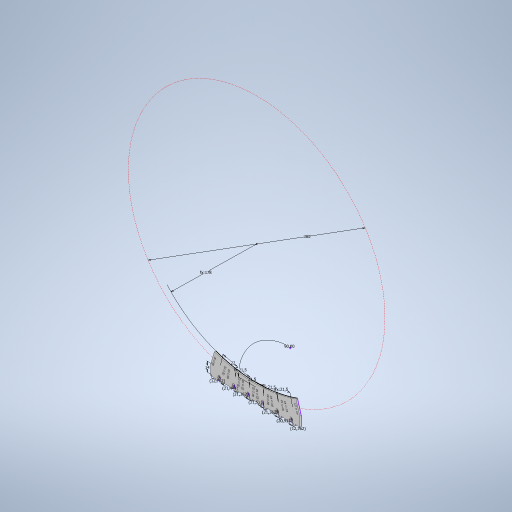
# Autodesk Inventor part: keywell_support-back
Saved by Autodesk Inventor 2024.1 (Build 281209000, 209)
## iProperties
Created: 2019-06-30
Part Number: keywell_support-back
Material: Acier inoxydable
Document SubType Name: Modeling
Designer: Thibault
Density: 8 g/cm^3
Appearance: Semi-poli
Mass: 13.686 g
Surface Area: 39.9351 cm^2
Volume: 1.71076 cm^3
kws_bp_anchor_dist1: 12,762 mm
kws_bp_anchor_dist2: 20,951 mm
kws_bp_anchor_dist3: 21,362 mm
kws_bp_anchor_dist4: 21,500 mm
kws_bp_anchor_dist5: 21,362 mm
kws_bp_anchor_dist6: 21,444 mm
kws_bp_anchor_dist7: 12,762 mm
Author: Thibault
Autodesk Inventor part; units mm, degrees
ref_plane "YZ Plane" through (0, 0, 0) normal (1, 0, 0) x (0, 1, 0)
ref_plane "XZ Plane" through (0, 0, 0) normal (0, 1, 0) x (-1, 0, 0)
ref_plane "XY Plane" through (0, 0, 0) normal (0, 0, 1) x (1, 0, 0)
sketch "Anchor (nut side)" plane through (0, 0, 0) normal (0, 0, 1) x (1, 0, 0)
  line L0 (11.1, 0) -> (9.1, 0)
  line L1 (9.1, 0) -> (9.1, -2)
  line L2 (9.1, -2) -> (9.9, -2)
  line L3 (9.9, -2) -> (9.9, -4)
  line L4 (6.2, -4) -> (6.2, -2)
  line L5 (6.2, -2) -> (7, -2)
  line L6 (7, -2) -> (7, 0)
  line L7 (7, 0) -> (5, 0)
  line L8 (2, 0) -> (2, 2)
  line L9 (2, 0) -> (3, 0) construction
  line L10 (2, 2) -> (5, 2)
  line L11 (5, 2) -> (5, 0)
  line L12 (11.1, 0) -> (11.1, 2)
  line L13 (11.1, 2) -> (14.1, 2)
  line L14 (14.1, 2) -> (14.1, 0)
  line L15 (0, 0) -> (2, 0)
  line L16 (14.1, 0) -> (16.1, 0)
  line L17 (6.2, -4) -> (7, -4)
  line L18 (9.9, -4) -> (9.1, -4)
  line L19 (7, -4) -> (7, -6.25)
  line L20 (9.1, -4) -> (9.1, -6.25)
  line L21 (7.25, -6.5) -> (8.05, -6.5)
  arc A0 (7, -6.25) -> (7.25, -6.5) centre (7.25, -6.25) ccw
  arc A1 (8.85, -6.5) -> (9.1, -6.25) centre (8.85, -6.25) ccw
  line L22 (8.05, -6.5) -> (8.85, -6.5)
  line L23 (8.05, -3.8983) -> (8.05, -9.959) construction
  point P0 (9.1321, -0.6227)
  point P1 (7, -6.5)
  point P2 (9.1, -6.5)
  dimension "d3" = 2
  dimension "d7" = 6.1
  dimension "d10" = 2
  dimension "d11" = 2
  dimension "d12" = 0.8
  dimension "d13" = 2
  dimension "d14" = 0.8
  dimension "d15" = 2.1
  dimension "d18" = 2
  dimension "d19" = 0.8
  dimension "d20" = 0.8
  dimension "d21" = 2.5
  dimension "d22" = 2.5
  dimension "d23" = 2.1
  dimension "d38" = 2
  dimension "d39" = 0.25
  dimension "d120" = 3
  measures "d3" distance of point (0, 0) L8.start
  measures "d7" distance of L7.end L0.start
  measures "d10" distance of L0.start L0.end
  measures "d11" distance of L0.end L1.end
  measures "d12" distance of L1.end L2.end
  measures "d13" distance of L2.end L3.end
  measures "d14" distance of L4.end L5.end
  measures "d15" distance of L6.end L0.end
  measures "d18" distance of L14.end point (16.1, 0)
  measures "d19" distance of L4.start L17.end
  measures "d20" distance of L3.end L18.end
  measures "d21" distance of L17.end point (7, -6.5)
  measures "d22" distance of L18.end point (9.1, -6.5)
  measures "d23" distance of L17.end L18.end
  measures "d38" distance of the line from the sketch origin of L10
  measures "d39" radius of A0
  measures "d120" distance of L8.end L10.end
sketch "Anchor (screw side)" plane through (0, 0, 0) normal (0, 0, 1) x (1, 0, 0)
  circle A0 centre (93.8994, 50.2542) radius 1.05
  line L0 (90.8494, 51.2542) -> (87.8494, 51.2542)
  line L1 (87.8494, 51.2542) -> (87.8494, 49.2542)
  line L2 (87.8494, 49.2542) -> (90.8494, 49.2542)
  line L3 (90.8494, 49.2542) -> (90.8494, 51.2542)
  line L4 (99.9494, 51.2542) -> (96.9494, 51.2542)
  line L5 (96.9494, 51.2542) -> (96.9494, 49.2542)
  line L6 (96.9494, 49.2542) -> (99.9494, 49.2542)
  line L7 (99.9494, 49.2542) -> (99.9494, 51.2542)
  line L8 (90.8494, 51.2542) -> (96.9494, 49.2542) construction
  line L9 (96.9494, 51.2542) -> (90.8494, 49.2542) construction
  line L10 (85.8494, 53.2542) -> (101.9494, 53.2542) construction
  line L11 (101.9494, 53.2542) -> (101.9494, 47.2542) construction
  line L12 (101.9494, 47.2542) -> (85.8494, 47.2542) construction
  line L13 (85.8494, 47.2542) -> (85.8494, 53.2542) construction
  point P0 (103.5798, 50.1132)
  dimension "d27" = 2.1
  dimension "d28" = 3
  dimension "d29" = 2
  dimension "slot_distance" = 6.1
  dimension "d34" = 2
  dimension "d35" = 2
  dimension "d36" = 2
  dimension "d37" = 2
  measures "d27" diameter of A0
  measures "d28" distance of L2.end L1.end
  measures "d29" distance of L1.end L0.end
  measures "slot_distance" distance between parallel lines of L5 L3
  measures "d34" distance between parallel lines of L0 L10
  measures "d35" distance between parallel lines of L12 L2
  measures "d36" distance between parallel lines of L11 L7
  measures "d37" distance between parallel lines of L13 L1
sketch "Screwless anchor (male)" plane through (0, 0, 0) normal (0, 0, 1) x (1, 0, 0)
  line L0 (2, 0) -> (2, 2)
  line L1 (2, 0) -> (3, 0) construction
  line L2 (2, 2) -> (5, 2)
  line L3 (5, 2) -> (5, 0)
  line L4 (11.1, 0) -> (11.1, 2)
  line L5 (11.1, 2) -> (14.1, 2)
  line L6 (14.1, 2) -> (14.1, 0)
  line L7 (0, 0) -> (2, 0)
  line L8 (14.1, 0) -> (16.1, 0)
  line L9 (5, 0) -> (11.1, 0)
  point P0 (9.1321, -0.6227)
  dimension "d81" = 2
  dimension "d83" = 6.1
  dimension "d92" = 2
  dimension "d100" = 2
  dimension "d119" = 3
  measures "d81" distance of L7.start L0.start
  measures "d83" distance of L3.end L4.start
  measures "d92" distance of L6.end L8.end
  measures "d100" distance between parallel lines of L7 L2
  measures "d119" distance of L0.end L2.end
sketch "Screwless anchor (female)" plane through (0, 0, 0) normal (0, 0, 1) x (1, 0, 0)
  line L0 (91.6814, 51.6592) -> (88.6814, 51.6592)
  line L1 (88.6814, 51.6592) -> (88.6814, 49.6592)
  line L2 (88.6814, 49.6592) -> (91.6814, 49.6592)
  line L3 (91.6814, 49.6592) -> (91.6814, 51.6592)
  line L4 (100.7814, 51.6592) -> (97.7814, 51.6592)
  line L5 (97.7814, 51.6592) -> (97.7814, 49.6592)
  line L6 (97.7814, 49.6592) -> (100.7814, 49.6592)
  line L7 (100.7814, 49.6592) -> (100.7814, 51.6592)
  line L8 (86.6814, 53.6592) -> (102.7814, 53.6592) construction
  line L9 (102.7814, 53.6592) -> (102.7814, 47.6592) construction
  line L10 (102.7814, 47.6592) -> (86.6814, 47.6592) construction
  line L11 (86.6814, 47.6592) -> (86.6814, 53.6592) construction
  point P0 (103.5798, 50.1132)
  dimension "d106" = 3
  dimension "d107" = 2
  dimension "d108" = 3
  dimension "d109" = 6.1
  dimension "d110" = 2
  dimension "d111" = 2
  dimension "d112" = 2
  dimension "d113" = 2
  measures "d106" distance of L2.end L1.end
  measures "d107" distance of L1.end L0.end
  measures "d108" distance of L6.end L5.end
  measures "d109" distance between parallel lines of L5 L3
  measures "d110" distance between parallel lines of L0 L8
  measures "d111" distance between parallel lines of L10 L2
  measures "d112" distance between parallel lines of L9 L7
  measures "d113" distance between parallel lines of L11 L1
sketch "Anchor" plane through (0, 0, 0) normal (0, 0, 1) x (1, 0, 0)
  line L0 (-55.868, -124.6471) -> (-43.768, -138.5471) construction
  line L1 (-43.768, -124.6471) -> (-55.868, -138.5471) construction
  line L2 (-49.818, -129.7478) -> (-49.818, -133.4207) construction
  circle A0 centre (-49.818, -123.6471) radius 1.05
  line L3 (-52.868, -122.6471) -> (-55.868, -122.6471)
  line L4 (-55.868, -122.6471) -> (-55.868, -124.6471)
  line L5 (-55.868, -124.6471) -> (-52.868, -124.6471)
  line L6 (-52.868, -124.6471) -> (-52.868, -122.6471)
  line L7 (-43.768, -122.6471) -> (-46.768, -122.6471)
  line L8 (-46.768, -122.6471) -> (-46.768, -124.6471)
  line L9 (-46.768, -124.6471) -> (-43.768, -124.6471)
  line L10 (-43.768, -124.6471) -> (-43.768, -122.6471)
  line L11 (-52.868, -122.6471) -> (-46.768, -124.6471) construction
  line L12 (-46.768, -122.6471) -> (-52.868, -124.6471) construction
  line L13 (-57.868, -120.6471) -> (-41.768, -120.6471) construction
  line L14 (-41.768, -120.6471) -> (-41.768, -126.6471) construction
  line L15 (-41.768, -126.6471) -> (-57.868, -126.6471) construction
  line L16 (-57.868, -126.6471) -> (-57.868, -120.6471) construction
  circle A1 centre (-49.818, -139.5471) radius 1.05
  line L17 (-52.868, -138.5471) -> (-55.868, -138.5471)
  line L18 (-55.868, -138.5471) -> (-55.868, -140.5471)
  line L19 (-55.868, -140.5471) -> (-52.868, -140.5471)
  line L20 (-52.868, -140.5471) -> (-52.868, -138.5471)
  line L21 (-43.768, -138.5471) -> (-46.768, -138.5471)
  line L22 (-46.768, -138.5471) -> (-46.768, -140.5471)
  line L23 (-46.768, -140.5471) -> (-43.768, -140.5471)
  line L24 (-43.768, -140.5471) -> (-43.768, -138.5471)
  line L25 (-52.868, -138.5471) -> (-46.768, -140.5471) construction
  line L26 (-46.768, -138.5471) -> (-52.868, -140.5471) construction
  line L27 (-57.868, -136.5471) -> (-41.768, -136.5471) construction
  line L28 (-41.768, -136.5471) -> (-41.768, -142.5471) construction
  line L29 (-41.768, -142.5471) -> (-57.868, -142.5471) construction
  line L30 (-57.868, -142.5471) -> (-57.868, -136.5471) construction
  point P0 (-66.8969, -206.6558)
  point P1 (-49.818, -123.6471)
  point P2 (-49.818, -139.5471)
  dimension "d161" = 13.9
sketch "Esquisse2" plane through (0, 0, 0) normal (0, 0, 1) x (1, 0, 0)
  circle A0 centre (0, 0) radius 190 construction
  arc A1 (-60.5742, -167.3761) -> (60.1317, -167.5356) centre (0, 0) ccw
  line L0 (-66.3196, -186.9369) -> (-60.5742, -167.3761)
  line L1 (49.6599, -105.5882) -> (49.6599, -111.3573) construction
  line L2 (65.8254, -187.1115) -> (65.8254, -200.9369)
  line L3 (-66.3196, -186.9369) -> (-66.3196, -200.9369)
  line L4 (-1.4727, -184.1617) -> (1.4714, -184.1617) construction
  line L5 (60.1317, -167.5356) -> (65.8254, -187.1115)
  line L6 (-61.6072, -200.9369) -> (-66.3196, -200.9369)
  line L7 (-45.5072, -200.9369) -> (-40.163, -200.9369)
  line L8 (-24.063, -200.9369) -> (-18.8006, -200.9369)
  line L9 (-2.7006, -200.9369) -> (2.6994, -200.9369)
  line L10 (18.7994, -200.9369) -> (24.0617, -200.9369)
  line L11 (40.1617, -200.9369) -> (45.0129, -200.9369)
  line L12 (61.1129, -200.9369) -> (65.8254, -200.9369)
  line L13 (-3.4694, -184.0486) -> (-18.0318, -195.3427) construction
  line L14 (-4.1541, -196.1292) -> (-17.3472, -183.2621) construction
  line L15 (-8.9042, -189.8002) -> (-12.5714, -189.5924) construction
  circle A2 centre (-2.8134, -190.1454) radius 1.05
  line L16 (-1.6424, -187.1569) -> (-1.4727, -184.1617)
  line L17 (-1.4727, -184.1617) -> (-3.4694, -184.0486)
  line L18 (-3.4694, -184.0486) -> (-3.6392, -187.0437)
  line L19 (-3.6392, -187.0437) -> (-1.6424, -187.1569)
  line L20 (-2.1573, -196.2423) -> (-1.9876, -193.2471)
  line L21 (-1.9876, -193.2471) -> (-3.9844, -193.134)
  line L22 (-3.9844, -193.134) -> (-4.1541, -196.1292)
  line L23 (-4.1541, -196.1292) -> (-2.1573, -196.2423)
  line L24 (-1.6424, -187.1569) -> (-3.9844, -193.134) construction
  line L25 (-1.9876, -193.2471) -> (-3.6392, -187.0437) construction
  line L26 (0.6373, -182.2781) -> (-0.2737, -198.3523) construction
  line L27 (-0.2737, -198.3523) -> (-6.2641, -198.0128) construction
  line L28 (-6.2641, -198.0128) -> (-5.3531, -181.9386) construction
  line L29 (-5.3531, -181.9386) -> (0.6373, -182.2781) construction
  circle A3 centre (-18.6879, -189.2458) radius 1.05
  line L30 (-17.5169, -186.2572) -> (-17.3472, -183.2621)
  line L31 (-17.3472, -183.2621) -> (-19.344, -183.1489)
  line L32 (-19.344, -183.1489) -> (-19.5137, -186.1441)
  line L33 (-19.5137, -186.1441) -> (-17.5169, -186.2572)
  line L34 (-18.0318, -195.3427) -> (-17.8621, -192.3475)
  line L35 (-17.8621, -192.3475) -> (-19.8589, -192.2343)
  line L36 (-19.8589, -192.2343) -> (-20.0286, -195.2295)
  line L37 (-20.0286, -195.2295) -> (-18.0318, -195.3427)
  line L38 (-17.5169, -186.2572) -> (-19.8589, -192.2343) construction
  line L39 (-17.8621, -192.3475) -> (-19.5137, -186.1441) construction
  line L40 (-15.2372, -181.3784) -> (-16.1482, -197.4526) construction
  line L41 (-16.1482, -197.4526) -> (-22.1386, -197.1131) construction
  line L42 (-22.1386, -197.1131) -> (-21.2276, -181.0389) construction
  line L43 (-21.2276, -181.0389) -> (-15.2372, -181.3784) construction
  line L44 (58.0467, -174.6897) -> (48.0791, -190.1902) construction
  line L45 (61.426, -186.3082) -> (44.6998, -178.5716) construction
  line L46 (54.8387, -181.9234) -> (51.3118, -182.9492) construction
  circle A4 centre (60.6966, -180.2197) radius 1.05
  line L47 (60.805, -177.0118) -> (59.9671, -174.1311)
  line L48 (59.9671, -174.1311) -> (58.0467, -174.6897)
  line L49 (58.0467, -174.6897) -> (58.8846, -177.5703)
  line L50 (58.8846, -177.5703) -> (60.805, -177.0118)
  line L51 (63.3464, -185.7497) -> (62.5086, -182.869)
  line L52 (62.5086, -182.869) -> (60.5882, -183.4276)
  line L53 (60.5882, -183.4276) -> (61.426, -186.3082)
  line L54 (61.426, -186.3082) -> (63.3464, -185.7497)
  line L55 (60.805, -177.0118) -> (60.5882, -183.4276) construction
  line L56 (62.5086, -182.869) -> (58.8846, -177.5703) construction
  line L57 (61.329, -171.6521) -> (65.8254, -187.1115) construction
  line L58 (65.8254, -187.1115) -> (60.0641, -188.7872) construction
  line L59 (60.0641, -188.7872) -> (55.5677, -173.3278) construction
  line L60 (55.5677, -173.3278) -> (61.329, -171.6521) construction
  circle A5 centre (45.4292, -184.6602) radius 1.05
  line L61 (45.5376, -181.4523) -> (44.6998, -178.5716)
  line L62 (44.6998, -178.5716) -> (42.7794, -179.1302)
  line L63 (42.7794, -179.1302) -> (43.6172, -182.0108)
  line L64 (43.6172, -182.0108) -> (45.5376, -181.4523)
  line L65 (48.0791, -190.1902) -> (47.2412, -187.3096)
  line L66 (47.2412, -187.3096) -> (45.3208, -187.8681)
  line L67 (45.3208, -187.8681) -> (46.1586, -190.7487)
  line L68 (46.1586, -190.7487) -> (48.0791, -190.1902)
  line L69 (45.5376, -181.4523) -> (45.3208, -187.8681) construction
  line L70 (47.2412, -187.3096) -> (43.6172, -182.0108) construction
  line L71 (46.0617, -176.0927) -> (50.558, -191.5521) construction
  line L72 (50.558, -191.5521) -> (44.7968, -193.2277) construction
  line L73 (44.7968, -193.2277) -> (40.3004, -177.7683) construction
  line L74 (40.3004, -177.7683) -> (46.0617, -176.0927) construction
  line L75 (-39.9855, -192.0548) -> (-24.2404, -182.4782) construction
  line L76 (-37.9404, -180.1289) -> (-26.2855, -194.4042) construction
  line L77 (-33.9357, -186.954) -> (-30.3156, -187.5748) construction
  circle A6 centre (-39.9486, -185.9229) radius 1.05
  line L78 (-41.4497, -188.76) -> (-41.9568, -191.7168)
  line L79 (-41.9568, -191.7168) -> (-39.9855, -192.0548)
  line L80 (-39.9855, -192.0548) -> (-39.4785, -189.098)
  line L81 (-39.4785, -189.098) -> (-41.4497, -188.76)
  line L82 (-39.9117, -179.7909) -> (-40.4187, -182.7477)
  line L83 (-40.4187, -182.7477) -> (-38.4475, -183.0858)
  line L84 (-38.4475, -183.0858) -> (-37.9404, -180.1289)
  line L85 (-37.9404, -180.1289) -> (-39.9117, -179.7909)
  line L86 (-41.4497, -188.76) -> (-38.4475, -183.0858) construction
  line L87 (-40.4187, -182.7477) -> (-39.4785, -189.098) construction
  line L88 (-44.266, -193.35) -> (-41.5449, -177.4816) construction
  line L89 (-41.5449, -177.4816) -> (-35.6312, -178.4957) construction
  line L90 (-35.6312, -178.4957) -> (-38.3523, -194.3641) construction
  line L91 (-38.3523, -194.3641) -> (-44.266, -193.35) construction
  circle A7 centre (-24.2774, -188.6102) radius 1.05
  line L92 (-25.7785, -191.4473) -> (-26.2855, -194.4042)
  line L93 (-26.2855, -194.4042) -> (-24.3143, -194.7422)
  line L94 (-24.3143, -194.7422) -> (-23.8072, -191.7854)
  line L95 (-23.8072, -191.7854) -> (-25.7785, -191.4473)
  line L96 (-24.2404, -182.4782) -> (-24.7475, -185.4351)
  line L97 (-24.7475, -185.4351) -> (-22.7762, -185.7731)
  line L98 (-22.7762, -185.7731) -> (-22.2692, -182.8163)
  line L99 (-22.2692, -182.8163) -> (-24.2404, -182.4782)
  line L100 (-25.7785, -191.4473) -> (-22.7762, -185.7731) construction
  line L101 (-24.7475, -185.4351) -> (-23.8072, -191.7854) construction
  line L102 (-28.5948, -196.0374) -> (-25.8736, -180.169) construction
  line L103 (-25.8736, -180.169) -> (-19.9599, -181.1831) construction
  line L104 (-19.9599, -181.1831) -> (-22.6811, -197.0515) construction
  line L105 (-22.6811, -197.0515) -> (-28.5948, -196.0374) construction
  line L106 (-61.9181, -186.1452) -> (-45.1715, -178.4529) construction
  line L107 (-58.5082, -174.5357) -> (-48.5815, -190.0625) construction
  line L108 (-55.3192, -181.7779) -> (-51.7951, -182.813) construction
  circle A8 centre (-61.1726, -180.0586) radius 1.05
  line L109 (-62.9916, -182.7032) -> (-63.8371, -185.5816)
  line L110 (-63.8371, -185.5816) -> (-61.9181, -186.1452)
  line L111 (-61.9181, -186.1452) -> (-61.0727, -183.2668)
  line L112 (-61.0727, -183.2668) -> (-62.9916, -182.7032)
  line L113 (-60.4271, -173.972) -> (-61.2725, -176.8504)
  line L114 (-61.2725, -176.8504) -> (-59.3536, -177.4141)
  line L115 (-59.3536, -177.4141) -> (-58.5082, -174.5357)
  line L116 (-58.5082, -174.5357) -> (-60.4271, -173.972)
  line L117 (-62.9916, -182.7032) -> (-59.3536, -177.4141) construction
  line L118 (-61.2725, -176.8504) -> (-61.0727, -183.2668) construction
  line L119 (-66.3196, -186.9369) -> (-61.7824, -171.4895) construction
  line L120 (-61.7824, -171.4895) -> (-56.0256, -173.1804) construction
  line L121 (-56.0256, -173.1804) -> (-60.5628, -188.6278) construction
  line L122 (-60.5628, -188.6278) -> (-66.3196, -186.9369) construction
  circle A9 centre (-45.9171, -184.5395) radius 1.05
  line L123 (-47.7361, -187.1841) -> (-48.5815, -190.0625)
  line L124 (-48.5815, -190.0625) -> (-46.6626, -190.6261)
  line L125 (-46.6626, -190.6261) -> (-45.8171, -187.7477)
  line L126 (-45.8171, -187.7477) -> (-47.7361, -187.1841)
  line L127 (-45.1715, -178.4529) -> (-46.017, -181.3313)
  line L128 (-46.017, -181.3313) -> (-44.0981, -181.8949)
  line L129 (-44.0981, -181.8949) -> (-43.2526, -179.0165)
  line L130 (-43.2526, -179.0165) -> (-45.1715, -178.4529)
  line L131 (-47.7361, -187.1841) -> (-44.0981, -181.8949) construction
  line L132 (-46.017, -181.3313) -> (-45.8171, -187.7477) construction
  line L133 (-51.0641, -191.4178) -> (-46.5268, -175.9703) construction
  line L134 (-46.5268, -175.9703) -> (-40.77, -177.6612) construction
  line L135 (-40.77, -177.6612) -> (-45.3073, -193.1087) construction
  line L136 (-45.3073, -193.1087) -> (-51.0641, -191.4178) construction
  line L137 (17.3459, -183.2622) -> (4.1528, -196.1292) construction
  line L138 (18.0305, -195.3428) -> (3.4682, -184.0486) construction
  line L139 (12.5958, -189.5911) -> (8.9286, -189.7989) construction
  circle A10 centre (18.6866, -189.2459) radius 1.05
  line L140 (19.5125, -186.1442) -> (19.3427, -183.149)
  line L141 (19.3427, -183.149) -> (17.3459, -183.2622)
  line L142 (17.3459, -183.2622) -> (17.5157, -186.2574)
  line L143 (17.5157, -186.2574) -> (19.5125, -186.1442)
  line L144 (20.0273, -195.2296) -> (19.8576, -192.2345)
  line L145 (19.8576, -192.2345) -> (17.8608, -192.3476)
  line L146 (17.8608, -192.3476) -> (18.0305, -195.3428)
  line L147 (18.0305, -195.3428) -> (20.0273, -195.2296)
  line L148 (19.5125, -186.1442) -> (17.8608, -192.3476) construction
  line L149 (19.8576, -192.2345) -> (17.5157, -186.2574) construction
  line L150 (21.2264, -181.0391) -> (22.1372, -197.1133) construction
  line L151 (22.1372, -197.1133) -> (16.1469, -197.4527) construction
  line L152 (16.1469, -197.4527) -> (15.236, -181.3785) construction
  line L153 (15.236, -181.3785) -> (21.2264, -181.0391) construction
  circle A11 centre (2.8121, -190.1455) radius 1.05
  line L154 (3.6379, -187.0438) -> (3.4682, -184.0486)
  line L155 (3.4682, -184.0486) -> (1.4714, -184.1617)
  line L156 (1.4714, -184.1617) -> (1.6411, -187.1569)
  line L157 (1.6411, -187.1569) -> (3.6379, -187.0438)
  line L158 (4.1528, -196.1292) -> (3.983, -193.134)
  line L159 (3.983, -193.134) -> (1.9862, -193.2471)
  line L160 (1.9862, -193.2471) -> (2.156, -196.2423)
  line L161 (2.156, -196.2423) -> (4.1528, -196.1292)
  line L162 (3.6379, -187.0438) -> (1.9862, -193.2471) construction
  line L163 (3.983, -193.134) -> (1.6411, -187.1569) construction
  line L164 (5.3519, -181.9386) -> (6.2627, -198.0128) construction
  line L165 (6.2627, -198.0128) -> (0.2723, -198.3523) construction
  line L166 (0.2723, -198.3523) -> (-0.6385, -182.2781) construction
  line L167 (-0.6385, -182.2781) -> (5.3519, -181.9386) construction
  line L168 (37.9392, -180.1292) -> (26.2842, -194.4043) construction
  line L169 (39.9842, -192.0551) -> (24.2392, -182.4784) construction
  line L170 (33.9345, -186.9542) -> (30.3143, -187.575) construction
  circle A12 centre (39.9474, -185.9231) radius 1.05
  line L171 (40.4175, -182.748) -> (39.9105, -179.7912)
  line L172 (39.9105, -179.7912) -> (37.9392, -180.1292)
  line L173 (37.9392, -180.1292) -> (38.4463, -183.086)
  line L174 (38.4463, -183.086) -> (40.4175, -182.748)
  line L175 (41.9555, -191.7171) -> (41.4484, -188.7603)
  line L176 (41.4484, -188.7603) -> (39.4772, -189.0983)
  line L177 (39.4772, -189.0983) -> (39.9842, -192.0551)
  line L178 (39.9842, -192.0551) -> (41.9555, -191.7171)
  line L179 (40.4175, -182.748) -> (39.4772, -189.0983) construction
  line L180 (41.4484, -188.7603) -> (38.4463, -183.086) construction
  line L181 (41.5437, -177.4819) -> (44.2647, -193.3503) construction
  line L182 (44.2647, -193.3503) -> (38.351, -194.3644) construction
  line L183 (38.351, -194.3644) -> (35.63, -178.496) construction
  line L184 (35.63, -178.496) -> (41.5437, -177.4819) construction
  circle A13 centre (24.2761, -188.6104) radius 1.05
  line L185 (24.7462, -185.4352) -> (24.2392, -182.4784)
  line L186 (24.2392, -182.4784) -> (22.268, -182.8164)
  line L187 (22.268, -182.8164) -> (22.775, -185.7733)
  line L188 (22.775, -185.7733) -> (24.7462, -185.4352)
  line L189 (26.2842, -194.4043) -> (25.7772, -191.4475)
  line L190 (25.7772, -191.4475) -> (23.8059, -191.7855)
  line L191 (23.8059, -191.7855) -> (24.313, -194.7424)
  line L192 (24.313, -194.7424) -> (26.2842, -194.4043)
  line L193 (24.7462, -185.4352) -> (23.8059, -191.7855) construction
  line L194 (25.7772, -191.4475) -> (22.775, -185.7733) construction
  line L195 (25.8724, -180.1692) -> (28.5934, -196.0375) construction
  line L196 (28.5934, -196.0375) -> (22.6798, -197.0516) construction
  line L197 (22.6798, -197.0516) -> (19.9587, -181.1832) construction
  line L198 (19.9587, -181.1832) -> (25.8724, -180.1692) construction
  line L199 (-56.6072, -200.9369) -> (-54.6072, -200.9369)
  line L200 (-54.6072, -200.9369) -> (-54.6072, -198.9369)
  line L201 (-54.6072, -198.9369) -> (-55.4072, -198.9369)
  line L202 (-55.4072, -198.9369) -> (-55.4072, -196.9369)
  line L203 (-51.7072, -196.9369) -> (-51.7072, -198.9369)
  line L204 (-51.7072, -198.9369) -> (-52.5072, -198.9369)
  line L205 (-52.5072, -198.9369) -> (-52.5072, -200.9369)
  line L206 (-52.5072, -200.9369) -> (-50.5072, -200.9369)
  line L207 (-47.5072, -200.9369) -> (-47.5072, -202.9369)
  line L208 (-47.5072, -200.9369) -> (-48.5072, -200.9369) construction
  line L209 (-47.5072, -202.9369) -> (-50.5072, -202.9369)
  line L210 (-50.5072, -202.9369) -> (-50.5072, -200.9369)
  line L211 (-56.6072, -200.9369) -> (-56.6072, -202.9369)
  line L212 (-56.6072, -202.9369) -> (-59.6072, -202.9369)
  line L213 (-59.6072, -202.9369) -> (-59.6072, -200.9369)
  line L214 (-45.5072, -200.9369) -> (-47.5072, -200.9369)
  line L215 (-59.6072, -200.9369) -> (-61.6072, -200.9369)
  line L216 (-51.7072, -196.9369) -> (-52.5072, -196.9369)
  line L217 (-55.4072, -196.9369) -> (-54.6072, -196.9369)
  line L218 (-52.5072, -196.9369) -> (-52.5072, -194.6869)
  line L219 (-54.6072, -196.9369) -> (-54.6072, -194.6869)
  line L220 (-52.7572, -194.4369) -> (-53.5572, -194.4369)
  arc A14 (-52.5072, -194.6869) -> (-52.7572, -194.4369) centre (-52.7572, -194.6869) ccw
  arc A15 (-54.3572, -194.4369) -> (-54.6072, -194.6869) centre (-54.3572, -194.6869) ccw
  line L221 (-53.5572, -194.4369) -> (-54.3572, -194.4369)
  line L222 (-53.5572, -197.0387) -> (-53.5572, -190.9779) construction
  line L223 (-35.163, -200.9369) -> (-33.163, -200.9369)
  line L224 (-33.163, -200.9369) -> (-33.163, -198.9369)
  line L225 (-33.163, -198.9369) -> (-33.963, -198.9369)
  line L226 (-33.963, -198.9369) -> (-33.963, -196.9369)
  line L227 (-30.263, -196.9369) -> (-30.263, -198.9369)
  line L228 (-30.263, -198.9369) -> (-31.063, -198.9369)
  line L229 (-31.063, -198.9369) -> (-31.063, -200.9369)
  line L230 (-31.063, -200.9369) -> (-29.063, -200.9369)
  line L231 (-26.063, -200.9369) -> (-26.063, -202.9369)
  line L232 (-26.063, -200.9369) -> (-27.063, -200.9369) construction
  line L233 (-26.063, -202.9369) -> (-29.063, -202.9369)
  line L234 (-29.063, -202.9369) -> (-29.063, -200.9369)
  line L235 (-35.163, -200.9369) -> (-35.163, -202.9369)
  line L236 (-35.163, -202.9369) -> (-38.163, -202.9369)
  line L237 (-38.163, -202.9369) -> (-38.163, -200.9369)
  line L238 (-24.063, -200.9369) -> (-26.063, -200.9369)
  line L239 (-38.163, -200.9369) -> (-40.163, -200.9369)
  line L240 (-30.263, -196.9369) -> (-31.063, -196.9369)
  line L241 (-33.963, -196.9369) -> (-33.163, -196.9369)
  line L242 (-31.063, -196.9369) -> (-31.063, -194.6869)
  line L243 (-33.163, -196.9369) -> (-33.163, -194.6869)
  line L244 (-31.313, -194.4369) -> (-32.113, -194.4369)
  arc A16 (-31.063, -194.6869) -> (-31.313, -194.4369) centre (-31.313, -194.6869) ccw
  arc A17 (-32.913, -194.4369) -> (-33.163, -194.6869) centre (-32.913, -194.6869) ccw
  line L245 (-32.113, -194.4369) -> (-32.913, -194.4369)
  line L246 (-32.113, -197.0387) -> (-32.113, -190.9779) construction
  line L247 (-13.8006, -200.9369) -> (-11.8006, -200.9369)
  line L248 (-11.8006, -200.9369) -> (-11.8006, -198.9369)
  line L249 (-11.8006, -198.9369) -> (-12.6006, -198.9369)
  line L250 (-12.6006, -198.9369) -> (-12.6006, -196.9369)
  line L251 (-8.9006, -196.9369) -> (-8.9006, -198.9369)
  line L252 (-8.9006, -198.9369) -> (-9.7006, -198.9369)
  line L253 (-9.7006, -198.9369) -> (-9.7006, -200.9369)
  line L254 (-9.7006, -200.9369) -> (-7.7006, -200.9369)
  line L255 (-4.7006, -200.9369) -> (-4.7006, -202.9369)
  line L256 (-4.7006, -200.9369) -> (-5.7006, -200.9369) construction
  line L257 (-4.7006, -202.9369) -> (-7.7006, -202.9369)
  line L258 (-7.7006, -202.9369) -> (-7.7006, -200.9369)
  line L259 (-13.8006, -200.9369) -> (-13.8006, -202.9369)
  line L260 (-13.8006, -202.9369) -> (-16.8006, -202.9369)
  line L261 (-16.8006, -202.9369) -> (-16.8006, -200.9369)
  line L262 (-2.7006, -200.9369) -> (-4.7006, -200.9369)
  line L263 (-16.8006, -200.9369) -> (-18.8006, -200.9369)
  line L264 (-8.9006, -196.9369) -> (-9.7006, -196.9369)
  line L265 (-12.6006, -196.9369) -> (-11.8006, -196.9369)
  line L266 (-9.7006, -196.9369) -> (-9.7006, -194.6869)
  line L267 (-11.8006, -196.9369) -> (-11.8006, -194.6869)
  line L268 (-9.9506, -194.4369) -> (-10.7506, -194.4369)
  arc A18 (-9.7006, -194.6869) -> (-9.9506, -194.4369) centre (-9.9506, -194.6869) ccw
  arc A19 (-11.5506, -194.4369) -> (-11.8006, -194.6869) centre (-11.5506, -194.6869) ccw
  line L269 (-10.7506, -194.4369) -> (-11.5506, -194.4369)
  line L270 (-10.7506, -197.0387) -> (-10.7506, -190.9779) construction
  line L271 (7.6994, -200.9369) -> (9.6994, -200.9369)
  line L272 (9.6994, -200.9369) -> (9.6994, -198.9369)
  line L273 (9.6994, -198.9369) -> (8.8994, -198.9369)
  line L274 (8.8994, -198.9369) -> (8.8994, -196.9369)
  line L275 (12.5994, -196.9369) -> (12.5994, -198.9369)
  line L276 (12.5994, -198.9369) -> (11.7994, -198.9369)
  line L277 (11.7994, -198.9369) -> (11.7994, -200.9369)
  line L278 (11.7994, -200.9369) -> (13.7994, -200.9369)
  line L279 (16.7994, -200.9369) -> (16.7994, -202.9369)
  line L280 (16.7994, -200.9369) -> (15.7994, -200.9369) construction
  line L281 (16.7994, -202.9369) -> (13.7994, -202.9369)
  line L282 (13.7994, -202.9369) -> (13.7994, -200.9369)
  line L283 (7.6994, -200.9369) -> (7.6994, -202.9369)
  line L284 (7.6994, -202.9369) -> (4.6994, -202.9369)
  line L285 (4.6994, -202.9369) -> (4.6994, -200.9369)
  line L286 (18.7994, -200.9369) -> (16.7994, -200.9369)
  line L287 (4.6994, -200.9369) -> (2.6994, -200.9369)
  line L288 (12.5994, -196.9369) -> (11.7994, -196.9369)
  line L289 (8.8994, -196.9369) -> (9.6994, -196.9369)
  line L290 (11.7994, -196.9369) -> (11.7994, -194.6869)
  line L291 (9.6994, -196.9369) -> (9.6994, -194.6869)
  line L292 (11.5494, -194.4369) -> (10.7494, -194.4369)
  arc A20 (11.7994, -194.6869) -> (11.5494, -194.4369) centre (11.5494, -194.6869) ccw
  arc A21 (9.9494, -194.4369) -> (9.6994, -194.6869) centre (9.9494, -194.6869) ccw
  line L293 (10.7494, -194.4369) -> (9.9494, -194.4369)
  line L294 (10.7494, -197.0387) -> (10.7494, -190.9779) construction
  line L295 (29.0617, -200.9369) -> (31.0617, -200.9369)
  line L296 (31.0617, -200.9369) -> (31.0617, -198.9369)
  line L297 (31.0617, -198.9369) -> (30.2617, -198.9369)
  line L298 (30.2617, -198.9369) -> (30.2617, -196.9369)
  line L299 (33.9617, -196.9369) -> (33.9617, -198.9369)
  line L300 (33.9617, -198.9369) -> (33.1617, -198.9369)
  line L301 (33.1617, -198.9369) -> (33.1617, -200.9369)
  line L302 (33.1617, -200.9369) -> (35.1617, -200.9369)
  line L303 (38.1617, -200.9369) -> (38.1617, -202.9369)
  line L304 (38.1617, -200.9369) -> (37.1617, -200.9369) construction
  line L305 (38.1617, -202.9369) -> (35.1617, -202.9369)
  line L306 (35.1617, -202.9369) -> (35.1617, -200.9369)
  line L307 (29.0617, -200.9369) -> (29.0617, -202.9369)
  line L308 (29.0617, -202.9369) -> (26.0617, -202.9369)
  line L309 (26.0617, -202.9369) -> (26.0617, -200.9369)
  line L310 (40.1617, -200.9369) -> (38.1617, -200.9369)
  line L311 (26.0617, -200.9369) -> (24.0617, -200.9369)
  line L312 (33.9617, -196.9369) -> (33.1617, -196.9369)
  line L313 (30.2617, -196.9369) -> (31.0617, -196.9369)
  line L314 (33.1617, -196.9369) -> (33.1617, -194.6869)
  line L315 (31.0617, -196.9369) -> (31.0617, -194.6869)
  line L316 (32.9117, -194.4369) -> (32.1117, -194.4369)
  arc A22 (33.1617, -194.6869) -> (32.9117, -194.4369) centre (32.9117, -194.6869) ccw
  arc A23 (31.3117, -194.4369) -> (31.0617, -194.6869) centre (31.3117, -194.6869) ccw
  line L317 (32.1117, -194.4369) -> (31.3117, -194.4369)
  line L318 (32.1117, -197.0387) -> (32.1117, -190.9779) construction
  line L319 (50.0129, -200.9369) -> (52.0129, -200.9369)
  line L320 (52.0129, -200.9369) -> (52.0129, -198.9369)
  line L321 (52.0129, -198.9369) -> (51.2129, -198.9369)
  line L322 (51.2129, -198.9369) -> (51.2129, -196.9369)
  line L323 (54.9129, -196.9369) -> (54.9129, -198.9369)
  line L324 (54.9129, -198.9369) -> (54.1129, -198.9369)
  line L325 (54.1129, -198.9369) -> (54.1129, -200.9369)
  line L326 (54.1129, -200.9369) -> (56.1129, -200.9369)
  line L327 (59.1129, -200.9369) -> (59.1129, -202.9369)
  line L328 (59.1129, -200.9369) -> (58.1129, -200.9369) construction
  line L329 (59.1129, -202.9369) -> (56.1129, -202.9369)
  line L330 (56.1129, -202.9369) -> (56.1129, -200.9369)
  line L331 (50.0129, -200.9369) -> (50.0129, -202.9369)
  line L332 (50.0129, -202.9369) -> (47.0129, -202.9369)
  line L333 (47.0129, -202.9369) -> (47.0129, -200.9369)
  line L334 (61.1129, -200.9369) -> (59.1129, -200.9369)
  line L335 (47.0129, -200.9369) -> (45.0129, -200.9369)
  line L336 (54.9129, -196.9369) -> (54.1129, -196.9369)
  line L337 (51.2129, -196.9369) -> (52.0129, -196.9369)
  line L338 (54.1129, -196.9369) -> (54.1129, -194.6869)
  line L339 (52.0129, -196.9369) -> (52.0129, -194.6869)
  line L340 (53.8629, -194.4369) -> (53.0629, -194.4369)
  arc A24 (54.1129, -194.6869) -> (53.8629, -194.4369) centre (53.8629, -194.6869) ccw
  arc A25 (52.2629, -194.4369) -> (52.0129, -194.6869) centre (52.2629, -194.6869) ccw
  line L341 (53.0629, -194.4369) -> (52.2629, -194.4369)
  line L342 (53.0629, -197.0387) -> (53.0629, -190.9779) construction
  point P0 (-32.113, -187.2665)
  point P1 (-53.5448, -182.2991)
  point P2 (10.7494, -189.6957)
  point P3 (32.1117, -187.2668)
  point P4 (-10.7506, -189.6956)
  point P5 (53.0629, -182.4399)
  point P6 (-53.5448, -182.2991)
  point P7 (-32.113, -187.2665)
  point P8 (-10.7506, -189.6956)
  point P9 (32.1117, -187.2668)
  point P10 (53.0629, -182.4399)
  point P11 (2.6994, -200.9369)
  point P12 (-59.9228, -201.5409)
  point P13 (53.0629, -182.4399)
  point P14 (32.1117, -187.2668)
  point P15 (10.7494, -189.6957)
  point P16 (-10.7506, -189.6956)
  point P17 (-32.113, -187.2665)
  point P18 (-53.5572, -182.2954)
  point P19 (43.8121, -201.5417)
  point P20 (49.6599, -108.4728)
  point P21 (22.268, -182.8164)
  dimension "kws_bp_anchor_dist2" = 20.9512
  dimension "kws_bp_anchor_dist3" = 21.3624
  dimension "kws_bp_anchor_dist4" = 21.5
  dimension "kws_bp_anchor_dist5" = 21.3623
  dimension "kws_bp_anchor_dist6" = 21.4442
  dimension "radius" = 380
  dimension "d73" = 178
  dimension "d163" = 22
  dimension "d164" = 21.5
  dimension "d165" = 21.5
  dimension "d166" = 21.5
  dimension "d167" = 21.5
  dimension "kws_bp_anchor_dist1" = 12.7625
  dimension "kws_bp_anchor_dist7" = 12.7625
  dimension "d196" = 14
  dimension "d200" = 90
  constraints: 26 end point, 8 point on circle, 7 horizontal, 3 vertical, 2 centre point, 1 coincident, 1 midpoint, 50 other
  measures "radius" diameter of A0
  measures "d73" radius of A1
  measures "d163" distance of A0.start A0.end
  measures "d164" distance of point (-10.751, -189.696) point (10.749, -189.696)
  measures "d165" distance of point (10.749, -189.696) point (32.112, -187.267)
  measures "d166" distance of point (32.112, -187.267) point (53.063, -182.44)
  measures "d167" distance of A0.start point (-10.751, -189.696)
  measures "d196" distance of L0.start L3.end
  measures "d200" angle of L1 L4
extrude "Base" add sketch "Esquisse2" along normal blind 2
sketch "Esquisse5" plane through (0, 0, 2) normal (0, 0, 1) x (1, 0, 0)
  line L0 (30.85, -115.1194) -> (153.5888, -115.1194)
  line L1 (153.5888, -115.1194) -> (153.5888, -267.9199)
  line L2 (30.85, -115.1194) -> (44.2647, -193.3503)
  line L3 (44.2647, -193.3503) -> (44.2647, -267.9199)
  line L4 (44.2647, -267.9199) -> (153.5888, -267.9199)
  line L5 (39.9105, -179.7912) -> (40.4175, -182.748) projected
  line L6 (41.9555, -191.7171) -> (39.9842, -192.0551) projected
  point P0 (0, 0)
  dimension "d171" = 2
  dimension "d172" = 2
  constraints: 10 end point, 2 perpendicular, 1 horizontal, 1 parallel, 1 vertical
  measures "d171" distance between parallel lines of L5 L2
  measures "d172" distance from line of L2.end L6
extrude "Front: substract" [suppressed]
sketch "Esquisse7" plane through (0, 0, 2) normal (0, 0, 1) x (1, 0, 0)
  line L0 (42.2935, -193.6883) -> (32.9332, -139.1019)
  line L1 (41.263, -187.6788) -> (41.4743, -188.9113)
  line L2 (-150.8128, -242.8864) -> (-114.6966, -101.4138)
  line L3 (-114.6966, -101.4138) -> (32.9332, -139.1019)
  line L4 (42.2935, -193.6883) -> (42.2935, -242.8864)
  line L5 (42.2935, -242.8864) -> (-150.8128, -242.8864)
  line L6 (43.6172, -182.0108) -> (42.7794, -179.1302) projected
  line L7 (39.9105, -179.7912) -> (40.4175, -182.748) projected
  line L8 (41.9555, -191.7171) -> (39.9842, -192.0551) projected
  point P0 (0, 0)
  dimension "d175" = 2
  constraints: 12 end point, 2 collinear, 2 perpendicular, 1 vertical
  measures "d175" distance from line of L0.start L8
extrude "Front r6: substract" [suppressed]
derived "shared_parameters.ipt"
sketch "Esquisse9" plane through (0, 0, 2) normal (0, 0, 1) x (1, 0, 0)
  line L0 (61.1129, -188.4822) -> (148.7656, -162.9883)
  line L1 (63.3464, -185.7497) -> (61.426, -186.3082) projected
  line L2 (61.1129, -188.4822) -> (61.1129, -267.18)
  line L3 (59.1129, -202.9369) -> (59.1129, -200.9369) projected
  line L4 (148.7656, -162.9883) -> (148.7656, -267.18)
  line L5 (148.7656, -267.18) -> (61.1129, -267.18)
  point P0 (0, 0)
  dimension "d192" = 2
  dimension "d193" = 2
  constraints: 9 end point, 2 vertical, 1 parallel, 1 perpendicular
  measures "d192" distance between parallel lines of L0 L1
  measures "d193" distance between parallel lines of L2 L3
extrude "Gain de place" [suppressed]
equation "\"esd\" = 0.1"
